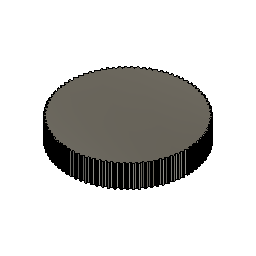
gear_85z (Autodesk Fusion 360 design; units mm, degrees)
Autodesk Fusion 360 part; units mm, degrees
sketch "Sketch1" plane through (0, 0, 0) normal (0, 0, 1) x (1, 0, 0) in component "gt2 pulley"
  circle A0 centre (0, 0) radius 27.0563 construction
  circle A1 centre (0, 0) radius 26.0523 construction
  line L0 (0, 0) -> (0, 27.0563) construction
  line L1 (0, 0) -> (0.9998, 27.0379) construction
  line L2 (0, 0) -> (1.4046, 27.0199) construction
  circle A2 centre (0, 0) radius 26.8023 construction
  arc A3 (0.3965, 26.6662) -> (0.474, 26.3684) centre (1.3915, 26.7662) ccw
  circle A4 centre (0, 0) radius 26.6523 construction
  arc A5 (0.2485, 26.8012) -> (0, 26.8023) centre (0, 0) ccw
  arc A6 (0.3965, 26.6662) -> (0.2485, 26.8012) centre (0.2472, 26.6512) ccw
  arc A7 (0.474, 26.3684) -> (0.9627, 26.0345) centre (0.9832, 26.5892) ccw
  arc A8 (0, 26.8023) -> (-0.2485, 26.8012) centre (0, 0) ccw
  arc A9 (-0.2485, 26.8012) -> (-0.3965, 26.6662) centre (-0.2472, 26.6512) ccw
  arc A10 (-0.474, 26.3684) -> (-0.3965, 26.6662) centre (-1.3915, 26.7662) ccw
  arc A11 (-0.9626, 26.0346) -> (-0.474, 26.3684) centre (-0.9832, 26.5892) ccw
  arc A12 (0.9627, 26.0345) -> (-0.9627, 26.0345) centre (0, 0) ccw
  point P0 (1.3915, 26.7662)
  point P1 (0, 26.8023)
  dimension "d18" = 54.1127
  dimension "d19" = 2.118
  dimension "d22" = 1.004
  dimension "d24" = 0.75
  dimension "d26" = 1
  dimension "d27" = 0.15
  dimension "d28" = 0.15
  dimension "d47" = 0.555
  dimension "d52" = 3.812
  constraint coincident A0.centre A1.centre
  constraint coincident A0 L0.end
  constraint vertical L0
  constraint coincident A0 L1.end
  constraint coincident A0 L2.end
  constraint concentric A1 A2
  constraint coincident A1 A7.end
  constraint coincident L1 A7.end
  constraint coincident A2 P0
  constraint coincident L2 P0
  constraint coincident P0 A3.centre
  constraint coincident A2 P1
  constraint coincident L0 P1
  constraint concentric A2 A4
  constraint coincident P1 A5.end
  constraint coincident A4 A6.centre
  constraint coincident A3.start A6.start
  constraint tangent A3 A6
  constraint tangent A3 A7
  constraint symmetric L0 A7.end A12.end
  constraint symmetric L0 A3.start A9.end
  constraint symmetric L0 A3.end A10.start
  constraint symmetric L0 A3 A10
  constraint symmetric L0 A5.start A8.end
  constraint symmetric L0 P1 A5.end
  constraint symmetric L0 A5 A8
  constraint symmetric L0 A6 A9
  constraint symmetric L0 A7 A11
  constraint coincident A1 A11.start
  constraint tangent A1 A7
  constraint coincident L1 A7.centre
  measures "d18" diameter of A0
  measures "d19" angle of L0 L1
  measures "d22" distance of A0 A1
  measures "d24" distance of A1 A2
  measures "d26" radius of A3
  measures "d27" distance of A2 A4
  measures "d28" radius of A6
  measures "d47" radius of A7
extrude "Extrude1" add sketch "Sketch1" along normal blind 10 makes body 1
pattern_circular "C-Pattern1" count 85 over 360 about axis through (0, 0, 1.75) along (0, 0, 1) of bodies 1 makes body 2 at (-1.1765, 26.0258, 3.3333) makes body 3 at (-3.9433, 25.7522, 6.6667) makes body 4 at (-4.9973, 25.5686, 3.3333) makes body 5 at (-6.8719, 25.1297, 3.3333) makes body 6 at (-8.709, 24.5536, 3.3333) makes body 7 at (-11.2761, 23.4856, 6.6667) makes body 8 at (-12.9798, 22.5887, 6.6667) makes body 9 at (-13.8962, 22.0368, 3.3333) makes body 10 at (-16.664, 20.0259, 6.6667) makes body 11 at (-16.9907, 19.7494, 3.3333) makes body 12 at (-19.2889, 17.5118, 6.6667) makes body 13 at (-19.7145, 17.0312, 3.3333) makes body 14 at (-21.7762, 14.3012, 6.6667) makes body 15 at (-22.0082, 13.9415, 3.3333) makes body 16 at (-23.6452, 10.9375, 6.6667) makes body 17 at (-24.1553, 9.7594, 6.6667) makes body 18 at (-24.9984, 7.3352, 6.6667) makes body 19 at (-25.3294, 6.0949, 6.6667) makes body 20 at (-25.7103, 4.2076, 6.6667) makes body 21 at (-25.9996, 1.6573, 6.6667) makes body 22 at (-26.051, -0.2674, 6.6667) makes body 23 at (-25.9601, -2.1906, 6.6667) makes body 24 at (-25.8207, -3.4667, 6.6667) makes body 25 at (-25.6565, -4.5239, 3.3333) makes body 26 at (-25.2524, -6.4064, 3.3333) makes body 27 at (-24.7103, -8.2538, 3.3333) makes body 28 at (-23.69, -10.8402, 6.6667) makes body 29 at (-23.2249, -11.8037, 3.3333) makes body 30 at (-22.2898, -13.4867, 3.3333) makes body 31 at (-21.2329, -15.096, 3.3333) makes body 32 at (-20.06, -16.6229, 3.3333) makes body 33 at (-17.709, -19.108, 6.6667) makes body 34 at (-17.3926, -19.3964, 3.3333) makes body 35 at (-14.7011, -21.5082, 6.6667) makes body 36 at (-13.6238, -22.2063, 6.6667) makes body 37 at (-11.3726, -23.439, 6.6667) makes body 38 at (-9.809, -24.1352, 6.6667) makes body 39 at (-8.406, -24.659, 6.6667) makes body 40 at (-7.3865, -24.9833, 3.3333) makes body 41 at (-4.682, -25.6282, 6.6667) makes body 42 at (-3.6258, -25.7988, 3.3333) makes body 43 at (-1.7106, -25.9961, 3.3333) makes body 44 at (1.7105, -25.9961, 6.6667) makes body 45 at (2.1373, -25.9645, 3.3333) makes body 46 at (4.0491, -25.7358, 3.3333) makes body 47 at (6.7686, -25.1577, 6.6667) makes body 48 at (7.7958, -24.8586, 3.3333) makes body 49 at (10.4006, -23.8862, 6.6667) makes body 50 at (11.3725, -23.4391, 6.6667) makes body 51 at (13.8056, -22.0937, 6.6667) makes body 52 at (14.701, -21.5082, 3.3333) makes body 53 at (16.2493, -20.3638, 3.3333) makes body 54 at (17.7089, -19.1081, 6.6667) makes body 55 at (20.06, -16.6229, 6.6667) makes body 56 at (21.2328, -15.0961, 6.6667) makes body 57 at (21.478, -14.7452, 3.3333) makes body 58 at (23.1272, -11.9941, 6.6667) makes body 59 at (23.4157, -11.4206, 3.3333) makes body 60 at (24.7103, -8.2539, 6.6667) makes body 61 at (25.0869, -7.0267, 6.6667) makes body 62 at (25.3542, -5.9907, 3.3333) makes body 63 at (25.8982, -2.8297, 6.6667) makes body 64 at (26.0431, -0.6954, 6.6667) makes body 65 at (26.0233, 1.2298, 6.6667) makes body 66 at (25.8614, 3.1483, 6.6667) makes body 67 at (25.5583, 5.0497, 6.6667) makes body 68 at (25.1716, 6.7169, 6.6667) makes body 69 at (24.744, 8.1522, 6.6667) makes body 70 at (24.3884, 9.1613, 3.3333) makes body 71 at (23.2732, 11.7082, 6.6667) makes body 72 at (22.0082, 13.9414, 6.6667) makes body 73 at (20.9185, 15.5287, 6.6667) makes body 74 at (19.8538, 16.8687, 6.6667) makes body 75 at (18.8516, 17.9817, 6.6667) makes body 76 at (18.0975, 18.7405, 3.3333) makes body 77 at (16.1656, 20.4303, 6.6667) makes body 78 at (13.8963, 22.0367, 6.6667) makes body 79 at (12.2309, 23.0028, 6.6667) makes body 80 at (11.8514, 23.2006, 3.3333) makes body 81 at (9.3114, 24.3315, 6.6667) makes body 82 at (7.489, 24.9527, 6.6667) makes body 83 at (6.4582, 25.2392, 3.3333) makes body 84 at (3.0954, 25.8678, 6.6667) makes body 85 at (1.8174, 25.9889, 6.6667)
sketch "Sketch2" plane through (0, 0, 10) normal (0, 0, 1) x (-1, 0, 0)
  arc A0 (-18.2579, -19.4395) -> (-18.2395, -19.6389) centre (-18.1375, -19.5289) ccw
  arc A1 (-18.2395, -19.6389) -> (-17.8722, -19.9738) centre (0, 0) ccw
  arc A2 (-17.8722, -19.9738) -> (-17.6719, -19.9737) centre (-17.7721, -19.862) ccw
  arc A3 (-17.414, -19.8058) -> (-17.6719, -19.9737) centre (-17.004, -20.7179) ccw
  arc A4 (-16.828, -19.8882) -> (-17.414, -19.8058) centre (-17.1864, -20.312) ccw
  arc A5 (-18.2508, -18.5912) -> (-16.828, -19.8882) centre (0, 0) ccw
  arc A6 (-18.1145, -19.1671) -> (-18.2508, -18.5912) centre (-18.6396, -18.9873) ccw
  arc A7 (-18.2579, -19.4395) -> (-18.1145, -19.1671) centre (-19.0606, -18.843) ccw
  circle A8 centre (0, 0) radius 26.0523
  constraint coincident A1.centre A5.centre
extrude "Extrude2" add sketch "Sketch2" against normal blind 10 contours A5 A8 bodies 1 2 3 4 5 6 7 8 9 10 11 12 13 14 15 16 17 18 19 20 21 22 23 24 25 26 27 28 29 30 31 32 33 34 35 36 37 38 39 40 41 42 43 44 45 46 47 48 49 50 51 52 53 54 55 56 57 58 59 60 61 62 63 64 65 66 67 68 69 70 71 72 73 74 75 76 77 78 79 80 81 82 83 84 85
extrude "Extrude4" [suppressed] in component "gt2 pulley"
pattern_circular "C-Pattern7" [suppressed] in component "gt2 pulley"
extrude "Extrude3" [suppressed] in component "gt2 pulley"
pattern_circular "C-Pattern6" [suppressed] in component "gt2 pulley"
extrude "Extrude2'" [suppressed] in component "gt2 pulley"
pattern_circular "C-Pattern5" [suppressed] in component "gt2 pulley"
extrude "Extrude1'" [suppressed] in component "gt2 pulley"
pattern_circular "C-Pattern4" [suppressed] in component "gt2 pulley"
pattern_circular "C-Pattern3" [suppressed] in component "gt2 pulley"
pattern_circular "C-Pattern2" [suppressed] in component "gt2 pulley"
pattern_circular "C-Pattern1'" [suppressed] in component "gt2 pulley"
copy_body "Body->Comp1" [suppressed] in component "Component"
copy_body "Body->Comp2" [suppressed] in component "Component'"
copy_body "Body->Comp3" [suppressed] in component "Component''"
copy_body "Body->Comp4" [suppressed] in component "Component'''"
copy_body "Body->Comp5" [suppressed] in component "Component''''"
copy_body "Body->Comp6" [suppressed] in component "Component'''''"
copy_body "Body->Comp7" [suppressed] in component "Component''''''"
copy_body "Body->Comp8" [suppressed] in component "Component'''''''"
copy_body "Body->Comp9" [suppressed] in component "Component''''''''"
copy_body "Body->Comp10" [suppressed] in component "Component'''''''''"
copy_body "Body->Comp11" [suppressed] in component "Component''''''''''"
copy_body "Body->Comp12" [suppressed] in component "Component'''''''''''"
copy_body "Body->Comp13" [suppressed] in component "Component''''''''''''"
copy_body "Body->Comp14" [suppressed] in component "Component'''''''''''''"
copy_body "Body->Comp15" [suppressed] in component "Component''''''''''''''"
copy_body "Body->Comp16" [suppressed] in component "Component'''''''''''''''"
copy_body "Body->Comp17" [suppressed] in component "Component''''''''''''''''"
copy_body "Body->Comp18" [suppressed] in component "Component'''''''''''''''''"
copy_body "Body->Comp19" [suppressed] in component "Component''''''''''''''''''"
copy_body "Body->Comp20" [suppressed] in component "Component'''''''''''''''''''"
component "gt2 pulley" placed x (1, 0, 0) y (0, 1, 0) z (0, 0, 1) at (0, 0, 0)
equation "NumTeeth = 85" comment "min 20"
equation "ToothPitch = 2 mm"
equation "PullyDia = NumTeeth * ToothPitch / PI"
equation "ToothAng = ( ( 360 / NumTeeth ) * 1 deg )"
equation "TransOffsetAngle = ToothAng * 0.2"
equation "Sholulder_Radius = 0.15 mm"
equation "Root_Radius = 0.555 mm"
equation "TransRadius = 1 mm"
equation "ToolHeight = 0.75 mm"
equation "PLD = 0.254 mm"
equation "d18 = PullyDia"
equation "d19 = ToothAng / 2"
equation "d22 = PLD + ToolHeight"
equation "d24 = ToolHeight"
equation "d26 = TransRadius"
equation "d27 = Sholulder_Radius"
equation "d31 = NumTeeth"
equation "d33 = NumTeeth"
equation "d35 = NumTeeth"
equation "d37 = NumTeeth"
equation "d41 = NumTeeth"
equation "d45 = NumTeeth"
equation "d47 = Root_Radius"
equation "d50 = NumTeeth"
